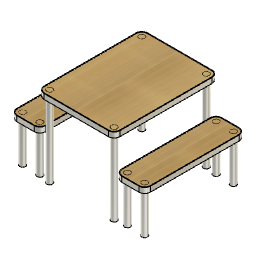
rgiro_quickcamp_table (Autodesk Fusion 360 design; units mm, degrees)
Autodesk Fusion 360 part; units mm, degrees
sketch "Sketch1" plane through (0, 0, 0) normal (0, 0, 1) x (1, 0, 0)
  line L0 (-330, -450) -> (330, -450)
  line L1 (330, -450) -> (330, 450)
  line L2 (330, 450) -> (-330, 450)
  line L3 (-330, 450) -> (-330, -450)
  line L4 (-330, -450) -> (330, 450) construction
  line L5 (330, -450) -> (-330, 450) construction
  circle A0 centre (-280, -400) radius 25
  circle A1 centre (-280, -400) radius 25
  circle A2 centre (280, -400) radius 25
  circle A3 centre (280, 400) radius 25
  circle A4 centre (-280, 400) radius 25
  line L6 (-580, -435) -> (-330, -435)
  line L7 (-330, -435) -> (-330, 435)
  line L8 (-330, 435) -> (-580, 435)
  line L9 (-580, 435) -> (-580, -435)
  line L10 (330, -435) -> (580, -435)
  line L11 (580, -435) -> (580, 435)
  line L12 (580, 435) -> (330, 435)
  line L13 (330, 435) -> (330, -435)
  circle A5 centre (-530, -385) radius 25
  circle A6 centre (-380, -385) radius 25
  circle A7 centre (-530, 385) radius 25
  circle A8 centre (-380, 385) radius 25
  circle A9 centre (380, -385) radius 25
  circle A10 centre (530, -385) radius 25
  circle A11 centre (530, 385) radius 25
  circle A12 centre (380, 385) radius 25
  dimension "d1" = 900
  dimension "d2" = 660
  dimension "d3" = 50
  dimension "d4" = 50
  dimension "d5" = 50
  dimension "d6" = 50
  dimension "d7" = 50
  dimension "d8" = 50
  dimension "d9" = 50
  dimension "d10" = 50
  dimension "d11" = 50
  dimension "d12" = 50
  dimension "d13" = 250
  dimension "d14" = 870
  dimension "d15" = 15
  dimension "d16" = 50
  dimension "d17" = 50
  dimension "d18" = 50
  dimension "d19" = 50
  dimension "d20" = 50
  dimension "d21" = 50
  dimension "d22" = 50
  dimension "d23" = 50
  dimension "d24" = 50
  dimension "d25" = 50
  dimension "d26" = 50
  dimension "d27" = 50
  dimension "d28" = 50
  dimension "d29" = 50
  dimension "d30" = 50
  dimension "d31" = 50
  constraint perpendicular L0 L1
  constraint parallel L0 L2
  constraint parallel L1 L3
  constraint horizontal L0
  constraint coincident L4 origin
  constraint coincident L5 origin
  constraint equal A1 A4
  constraint equal A0 A2
  constraint equal A0 A3
  constraint horizontal L6
  constraint vertical L7
  constraint horizontal L8
  constraint vertical L9
  constraint horizontal L10
  constraint vertical L11
  constraint horizontal L12
  constraint vertical L13
  constraint equal L9 L13
  constraint equal L6 L10
  constraint collinear L3 L7
  constraint collinear L1 L13
  constraint collinear L6 L10
  constraint equal A0 A9
  constraint equal A9 A10
  constraint equal A9 A11
  constraint equal A9 A12
  constraint equal A1 A8
  constraint equal A7 A8
  constraint equal A5 A7
  constraint equal A5 A6
  measures "d1" distance of L0.start L2.end
  measures "d2" distance of L0.start L0.end
  measures "d3" diameter of A0
  measures "d4" distance of L0 A0.centre
  measures "d5" distance of L3 A0.centre
  measures "d6" diameter of A1
  measures "d7" distance of L0 A2.centre
  measures "d8" distance of L2 A3.centre
  measures "d9" distance of L2 A4.centre
  measures "d10" distance of L3 A4.centre
  measures "d11" distance of L1 A3.centre
  measures "d12" distance of L1 A2.centre
  measures "d13" distance of L6.start L6.end
  measures "d14" distance of L6.start L8.end
  measures "d15" distance of L0 L6
  measures "d16" distance of L6 A5.centre
  measures "d17" distance of L9 A5.centre
  measures "d18" distance of L7 A6.centre
  measures "d19" distance of L6 A6.centre
  measures "d20" distance of L8 A8.centre
  measures "d21" distance of L8 A7.centre
  measures "d22" distance of L9 A7.centre
  measures "d23" distance of L7 A8.centre
  measures "d24" distance of L12 A11.centre
  measures "d25" distance of L12 A12.centre
  measures "d26" distance of L10 A9.centre
  measures "d27" distance of L10 A10.centre
  measures "d28" distance of L13 A9.centre
  measures "d29" distance of L11 A10.centre
  measures "d30" distance of L11 A11.centre
  measures "d31" distance of L13 A12.centre
extrude "Extrude1" add sketch "Sketch1" along normal blind 395 contours A5 | A6 | A7 | A8 | A9 | A10 | A11 | A12 makes body 1 at (-525.6588, -360.3798, 263.3333) makes body 2 at (404.9689, -386.2461, 263.3333) makes body 3 at (534.3412, 409.6202, 263.3333) makes body 4 at (-525.6588, 409.6202, 263.3333) makes body 5 at (-355.0311, -386.2461, 263.3333) makes body 6 at (534.3412, -360.3798, 263.3333) makes body 7 at (404.9689, 383.7539, 263.3333) makes body 8 at (-355.0311, 383.7539, 263.3333)
extrude "Extrude2" add sketch "Sketch1" along normal blind 695 separate body contours A0 A1 | A2 | A3 | A4 makes body 9 at (304.8758, 397.5108, 231.6667) makes body 10 at (304.8758, -402.4892, 231.6667) makes body 11 at (-255.1242, 397.5108, 231.6667) makes body 12 at (-255.1242, -402.4892, 231.6667)
sketch "Sketch2" plane through (0, 0, 395) normal (0, 0, 1) x (-1, 0, 0)
  circle A0 centre (530, -385) radius 25
  line L0 (-330, -435) -> (-330, 435)
  line L1 (-580, -435) -> (-330, -435)
  line L2 (-580, 435) -> (-580, -435)
  line L3 (-330, 435) -> (-580, 435)
  line L4 (330, 435) -> (330, -435)
  line L5 (330, -435) -> (580, -435)
  line L6 (580, -435) -> (580, 435)
  line L7 (580, 435) -> (330, 435)
extrude "Extrude3" add sketch "Sketch2" along normal blind 5 separate body contours A0 | L0 L1 L2 L3 | L4 L5 L6 L7 makes body 13 at (413.3333, 145, 395) makes body 14 at (-413.3333, -145, 395)
sketch "Sketch3" plane through (0, 0, 695) normal (0, 0, 1) x (-1, 0, 0)
  circle A0 centre (-280, -400) radius 25
  line L0 (330, 450) -> (-330, 450)
  line L1 (-330, -450) -> (330, -450)
  line L2 (330, -450) -> (330, 450)
  line L3 (-330, 450) -> (-330, -450)
extrude "Extrude4" add sketch "Sketch3" along normal blind 5 separate body contours A0 | L0 L1 L2 L3 makes body 15
fillet "Fillet2" radius 50 4 edges at (330, -450, 697.5) (-330, -450, 697.5) (-330, 450, 697.5) (330, 450, 697.5) on bodies 15
fillet "Fillet3" radius 50 4 edges at (580, 435, 397.5) (330, 435, 397.5) (580, -435, 397.5) (330, -435, 397.5) on bodies 13
fillet "Fillet4" radius 50 4 edges at (-580, -435, 397.5) (-330, -435, 397.5) (-580, 435, 397.5) (-330, 435, 397.5) on bodies 14
sketch "Sketch7" plane through (0, 0, 695) normal (0, 0, -1) x (1, 0, 0)
  arc A0 (280, -450) -> (330, -400) centre (280, -400) ccw
  line L0 (330, -400) -> (330, 400)
  arc A1 (330, 400) -> (280, 450) centre (280, 400) ccw
  line L1 (280, 450) -> (-280, 450)
  arc A2 (-280, 450) -> (-330, 400) centre (-280, 400) ccw
  line L2 (-330, 400) -> (-330, -400)
  arc A3 (-330, -400) -> (-280, -450) centre (-280, -400) ccw
  line L3 (-280, -450) -> (280, -450)
  arc A4 (280, -445) -> (325, -400) centre (280, -400) ccw
  line L4 (325, -400) -> (325, 400)
  arc A5 (325, 400) -> (280, 445) centre (280, 400) ccw
  line L5 (280, 445) -> (-280, 445)
  arc A6 (-280, 445) -> (-325, 400) centre (-280, 400) ccw
  line L6 (-325, 400) -> (-325, -400)
  arc A7 (-325, -400) -> (-280, -445) centre (-280, -400) ccw
  line L7 (-280, -445) -> (280, -445)
  dimension "d51" = -5
sketch "Sketch8" plane through (0, 0, 395) normal (0, 0, -1) x (1, 0, 0)
  arc A0 (-380, -435) -> (-330, -385) centre (-380, -385) ccw
  line L0 (-330, -385) -> (-330, 385)
  arc A1 (-330, 385) -> (-380, 435) centre (-380, 385) ccw
  line L1 (-380, 435) -> (-530, 435)
  arc A2 (-530, 435) -> (-580, 385) centre (-530, 385) ccw
  line L2 (-580, 385) -> (-580, -385)
  arc A3 (-580, -385) -> (-530, -435) centre (-530, -385) ccw
  line L3 (-530, -435) -> (-380, -435)
  line L4 (-335, -385) -> (-335, 385)
  arc A4 (-335, 385) -> (-380, 430) centre (-380, 385) ccw
  line L5 (-380, 430) -> (-530, 430)
  arc A5 (-530, 430) -> (-575, 385) centre (-530, 385) ccw
  line L6 (-575, 385) -> (-575, -385)
  arc A6 (-575, -385) -> (-530, -430) centre (-530, -385) ccw
  line L7 (-530, -430) -> (-380, -430)
  arc A7 (-380, -430) -> (-335, -385) centre (-380, -385) ccw
  dimension "d52" = -5
sketch "Sketch9" plane through (0, 0, 395) normal (0, 0, -1) x (1, 0, 0)
  arc A0 (380, 435) -> (330, 385) centre (380, 385) ccw
  line L0 (330, 385) -> (330, -385)
  arc A1 (330, -385) -> (380, -435) centre (380, -385) ccw
  line L1 (380, -435) -> (530, -435)
  arc A2 (530, -435) -> (580, -385) centre (530, -385) ccw
  line L2 (580, -385) -> (580, 385)
  arc A3 (580, 385) -> (530, 435) centre (530, 385) ccw
  line L3 (530, 435) -> (380, 435)
  line L4 (575, -385) -> (575, 385)
  arc A4 (575, 385) -> (530, 430) centre (530, 385) ccw
  line L5 (530, 430) -> (380, 430)
  arc A5 (380, 430) -> (335, 385) centre (380, 385) ccw
  line L6 (335, 385) -> (335, -385)
  arc A6 (335, -385) -> (380, -430) centre (380, -385) ccw
  line L7 (380, -430) -> (530, -430)
  arc A7 (530, -430) -> (575, -385) centre (530, -385) ccw
  dimension "d53" = -5
extrude "Extrude7" add sketch "Sketch7" along normal blind 45 separate body makes body 16
extrude "Extrude8" add sketch "Sketch9" along normal blind 45 separate body makes body 17
extrude "Extrude9" add sketch "Sketch8" along normal blind 45 separate body makes body 18
